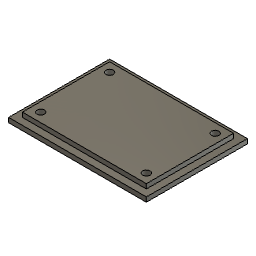
RGB LED Strip Housing Bottom v2 (Autodesk Fusion 360 design; units mm, degrees)
Autodesk Fusion 360 part; units mm, degrees
sketch "Sketch1" plane through (0, 0, 0) normal (0, 1, 0) x (1, 0, 0)
  line L0 (0, 0) -> (60, 0)
  line L1 (60, 0) -> (60, 44)
  line L2 (60, 44) -> (0, 44)
  line L3 (0, 44) -> (0, 0)
  line L4 (3, 41) -> (57, 41)
  line L5 (57, 41) -> (57, 3)
  line L6 (57, 3) -> (3, 3)
  line L7 (3, 3) -> (3, 41)
  circle A0 centre (7, 37) radius 1.6
  circle A1 centre (53, 37) radius 1.6
  line L8 (3, 22) -> (57, 22)
  circle A2 centre (7, 7) radius 1.6
  circle A3 centre (53, 7) radius 1.6
  dimension "d1" = 60
  dimension "d2" = 44
  dimension "d3" = 54
  dimension "d4" = 38
  dimension "d9" = 3.2
  dimension "d10" = 3.2
  constraint horizontal L0
  constraint vertical L1
  constraint horizontal L2
  constraint vertical L3
  constraint coincident L0.start L3.end
  constraint horizontal L4
  constraint vertical L5
  constraint horizontal L6
  constraint vertical L7
  constraint perpendicular L7 L8
  constraint midpoint L7 L8.start
  constraint midpoint L5 L8.end
  constraint symmetric A0 L8 A2
  constraint symmetric A1 L8 A3
  measures "d1" distance of L0.start L0.end
  measures "d2" distance of L0.start L2.end
  measures "d3" distance of L4.start L4.end
  measures "d4" distance of L4.start L6.end
  measures "d9" diameter of A0
  measures "d10" diameter of A1
extrude "Extrude1" add sketch "Sketch1" against normal blind 2 contours L0 L1 L2 L3 | L4 L5 L7 L8 | L5 L6 L7 L8 | A0 | A1 | A2 | A3
extrude "Extrude2" add sketch "Sketch1" along normal blind 2 contours L4 L5 L7 L8 | L5 L6 L7 L8 | A0 | A1 | A2 | A3
extrude "Extrude3" cut sketch "Sketch1" along normal blind 3 contours A0 | A1 | A2 | A3
extrude "Extrude4" cut sketch "Sketch1" against normal blind 8 contours A0 | A1 | A2 | A3
chamfer "Chamfer1" distance 0.75 angle 45 4 edges at (5.5083, -2, -6.4214) (5.5083, -2, -36.4214) (51.5083, -2, -36.4214) (51.5083, -2, -6.4214)
delete_face "DeleteFace1" 1 faces at (54.892, -1.75, -6.0888)
delete_face "DeleteFace2" 1 faces at (54.892, -1.75, -36.0888)
delete_face "DeleteFace3" 1 faces at (8.05, -1.75, -8.8187)
delete_face "DeleteFace4" 1 faces at (5.2649, -1.75, -38.183)
chamfer "Chamfer2" distance 1.5 angle 45 4 edges at (5.5083, -2, -7.5786) (51.5083, -2, -7.5786) (51.5083, -2, -37.5786) (5.5083, -2, -37.5786)
equation "d3 = 118 mm - 64 mm"
